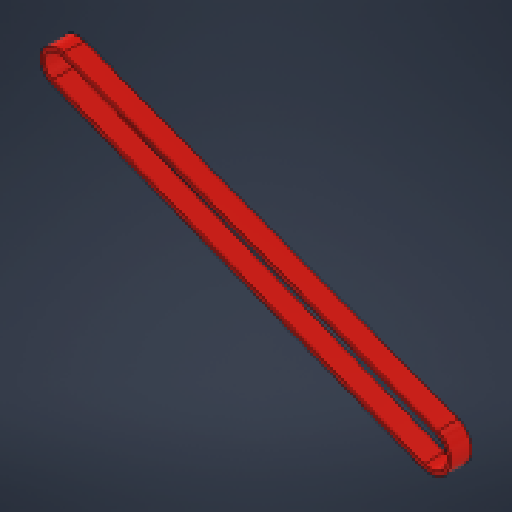
# Autodesk Inventor part: Single Indexer tensioner band
Saved by Autodesk Inventor 2023.2 (Build 272271030, 271C)
## iProperties
Created: 2023-04-07
Part Number: Single Indexer tensioner band
Material: Generic
Document SubType Name: Modeling
Designer: Main Account
Density: 1 g/cm^3
Appearance: Default
Author: Main Account
Autodesk Inventor part; units mm, degrees
ref_plane "YZ Plane" through (0, 0, 0) normal (1, 0, 0) x (0, 1, 0)
ref_plane "XZ Plane" through (0, 0, 0) normal (0, 1, 0) x (-1, 0, 0)
ref_plane "XY Plane" through (0, 0, 0) normal (0, 0, 1) x (1, 0, 0)
sketch "Sketch1" plane through (0, 0, 0) normal (0, 0, 1) x (1, 0, 0)
  circle A0 centre (13.2768, 2.5077) radius 4.064 construction
  circle A1 centre (-76.1973, 37.0416) radius 3.9624 construction
  arc A2 (-75.0816, 40.0141) -> (-77.3679, 34.0903) centre (-76.1973, 37.0416) ccw
  line L0 (-75.0816, 40.0141) -> (14.7049, 6.3125)
  line L1 (11.7784, -1.27) -> (-77.3679, 34.0903)
  arc A3 (11.7784, -1.27) -> (14.7049, 6.3125) centre (13.2768, 2.5077) ccw
  line L2 (15.0564, 7.2487) -> (-74.7302, 40.9503)
  arc A4 (-74.7302, 40.9503) -> (-77.7367, 33.1608) centre (-76.1973, 37.0416) ccw
  line L3 (-77.7367, 33.1608) -> (11.4097, -2.1995)
  arc A5 (11.4097, -2.1995) -> (15.0564, 7.2487) centre (13.2768, 2.5077) ccw
  point P0 (0, 0)
  dimension "d0" = 6.35
  dimension "d1" = 1
  constraints: 10 point on circle, 8 end point, 4 centre point, 4 tangent, 2 coincident, 1 concentric, 3 other
  measures "d0" diameter of A2
  measures "d1" distance between parallel lines of L0 L2
extrude "Extrusion1" add sketch "Sketch1" against normal blind 5
body "Solid1"
